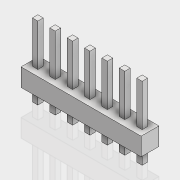
# Autodesk Inventor part: ЛЦМК.00002.00.00.00.00.01
Saved by Autodesk Inventor 2021.2 (Build 252289000, 289)
## iProperties
Created: 2025-10-22
Part Number: ЛЦМК.00002.00.00.00.00.01
Material: Типовые
Document SubType Name: Modeling
Designer: Захаров
Density: 1 g/cm^3
Appearance: По умолчанию
Author: Захаров
Autodesk Inventor part; units mm, degrees
ref_plane "YZ Plane" through (0, 0, 0) normal (1, 0, 0) x (0, 1, 0)
ref_plane "XZ Plane" through (0, 0, 0) normal (0, 1, 0) x (-1, 0, 0)
ref_plane "XY Plane" through (0, 0, 0) normal (0, 0, 1) x (1, 0, 0)
sketch "Эскиз1" plane through (0, 0, 0) normal (0, 0, 1) x (1, 0, 0)
  line L0 (8.75, -1.3) -> (-8.75, -1.3)
  line L1 (-8.75, -1.3) -> (-8.75, 1.3)
  line L2 (-8.75, 1.3) -> (8.75, 1.3)
  line L3 (8.75, 1.3) -> (8.75, -1.3)
  line L4 (8.75, -1.3) -> (-8.75, 1.3) construction
  line L5 (-8.75, -1.3) -> (8.75, 1.3) construction
  line L6 (-8, 7.4) -> (-7.2, 7.4)
  line L7 (-7.2, 7.4) -> (-7.2, 1.3)
  line L8 (-7.2, 1.3) -> (-8, 1.3)
  line L9 (-8, 1.3) -> (-8, 7.4)
  line L10 (-8, 1.3) -> (-7.2, 1.3)
  line L11 (-7.2, -3.2) -> (-8, -3.2)
  line L12 (-7.2, -1.3) -> (-7.2, -3.2)
  line L13 (-8, -3.2) -> (-8, -1.3)
  line L14 (-4.6667, 7.4) -> (-4.6667, 1.3)
  line L15 (-5.4667, 1.3) -> (-5.4667, 7.4)
  line L16 (-5.4667, 7.4) -> (-4.6667, 7.4)
  line L17 (-5.4667, -3.2) -> (-5.4667, -1.3)
  line L18 (-4.6667, -1.3) -> (-4.6667, -3.2)
  line L19 (-4.6667, -3.2) -> (-5.4667, -3.2)
  line L20 (-2.1333, 7.4) -> (-2.1333, 1.3)
  line L21 (-2.9333, 1.3) -> (-2.9333, 7.4)
  line L22 (-2.9333, 7.4) -> (-2.1333, 7.4)
  line L23 (-2.9333, -3.2) -> (-2.9333, -1.3)
  line L24 (-2.1333, -1.3) -> (-2.1333, -3.2)
  line L25 (-2.1333, -3.2) -> (-2.9333, -3.2)
  line L26 (0.4, 7.4) -> (0.4, 1.3)
  line L27 (-0.4, 1.3) -> (-0.4, 7.4)
  line L28 (-0.4, 7.4) -> (0.4, 7.4)
  line L29 (-0.4, -3.2) -> (-0.4, -1.3)
  line L30 (0.4, -1.3) -> (0.4, -3.2)
  line L31 (0.4, -3.2) -> (-0.4, -3.2)
  line L32 (2.9333, 7.4) -> (2.9333, 1.3)
  line L33 (2.1333, 1.3) -> (2.1333, 7.4)
  line L34 (2.1333, 7.4) -> (2.9333, 7.4)
  line L35 (2.1333, -3.2) -> (2.1333, -1.3)
  line L36 (2.9333, -1.3) -> (2.9333, -3.2)
  line L37 (2.9333, -3.2) -> (2.1333, -3.2)
  line L38 (5.4667, 7.4) -> (5.4667, 1.3)
  line L39 (4.6667, 1.3) -> (4.6667, 7.4)
  line L40 (4.6667, 7.4) -> (5.4667, 7.4)
  line L41 (4.6667, -3.2) -> (4.6667, -1.3)
  line L42 (5.4667, -1.3) -> (5.4667, -3.2)
  line L43 (5.4667, -3.2) -> (4.6667, -3.2)
  line L44 (8, 7.4) -> (8, 1.3)
  line L45 (7.2, 1.3) -> (7.2, 7.4)
  line L46 (7.2, 7.4) -> (8, 7.4)
  line L47 (7.2, -3.2) -> (7.2, -1.3)
  line L48 (8, -1.3) -> (8, -3.2)
  line L49 (8, -3.2) -> (7.2, -3.2)
  point P0 (0, 0)
  point P1 (-7.6, 1.3)
  point P2 (-4.6667, 1.3)
  point P3 (-2.1333, 1.3)
  point P4 (0.4, 1.3)
  point P5 (8, 1.3)
  point P6 (2.9333, 1.3)
  point P7 (5.4667, 1.3)
  point P8 (-7.2, 1.3)
  dimension "d0" = 17.5
  dimension "d1" = 2.6
  dimension "d3" = 8.7
  dimension "d7" = 4.5
  dimension "d8" = 0.75
  dimension "d9" = 0.8
  dimension "d12" = 2.5333
  constraints: 100 end point, 6 parallel, 4 horizontal, 3 midpoint, 3 perpendicular, 3 point on line, 1 collinear, 83 other
  measures "d0" distance of L1.end L2.end
  measures "d1" distance of L0.end L1.end
  measures "d3" distance between parallel lines of L6 L0
  measures "d7" distance between parallel lines of L2 L11
  measures "d8" horizontal distance of L0.end L11.end
  measures "d9" distance of L6.start L6.end
  measures "d12" distance of L6.end L14.start
extrude "Выдавливание1" add sketch "Эскиз1" against normal mid plane 2.6 contours L0 L1 L2 L3
extrude "Выдавливание2" add sketch "Эскиз1" along normal mid plane 0.8 contours L48 L49 L47 L0 | L2 L45 L46 L44 | L42 L43 L41 L0 | L2 L39 L40 L38 | L36 L37 L35 L0 | L2 L33 L34 L32 | L30 L31 L29 L0 | L2 L27 L28 L26 | L24 L25 L23 L0 | L2 L21 L22 L20 | L18 L19 L17 L0 | L2 L15 L16 L14 | L12 L11 L13 L0 | L2 L9 L6 L7
